Autodesk Fusion 360 part; units mm, degrees
note: some values were not read from the file. Chosen so that the rebuilt part matches the saved one: which bodies a step acts on. Set by a fixed rule: which sketch regions a step uses.
(part 2 of 5)
  constraint midpoint L119 L120.start
  constraint midpoint L117 L120.end
  constraint coincident L121 L124.start
  constraint coincident L122 L124.end
  constraint perpendicular L122 L124
  constraint midpoint L110 L169.start
  constraint midpoint L112 L169.end
  constraint symmetric A3.start L169 L12.end
  constraint symmetric L3.end L169 L11.end
  constraint symmetric L4.end L169 L10.end
  constraint symmetric L5.end L169 A8.start
  constraint symmetric L116.start L169 L170.end
  constraint symmetric L116.end L169 L173.start
  constraint symmetric L117.end L169 L172.start
  constraint symmetric L118.end L169 L170.start
  constraint symmetric L120.start L169 L171.start
  constraint symmetric L120.end L169 L171.end
  constraint symmetric L124.start L169 L218.start
  constraint symmetric L124.end L169 L218.end
  constraint symmetric L125.start L169 L176.start
  constraint symmetric L125.end L169 L176.end
  constraint symmetric L126.start L169 L175.start
  constraint symmetric L126.end L169 L174.start
  constraint symmetric L127.end L169 L174.end
  constraint symmetric L128.start L169 L180.start
  constraint symmetric L128.end L169 L180.end
  constraint symmetric L129.start L169 L179.start
  constraint symmetric L129.end L169 L178.start
  constraint symmetric L130.end L169 L178.end
  constraint symmetric L131.start L169 L184.start
  constraint symmetric L131.end L169 L184.end
  constraint symmetric L132.start L169 L183.start
  constraint symmetric L132.end L169 L182.start
  constraint symmetric L133.end L169 L182.end
  constraint symmetric L134.start L169 L188.start
  constraint symmetric L134.end L169 L188.end
  constraint symmetric L135.start L169 L187.start
  constraint symmetric L135.end L169 L186.start
  constraint symmetric L136.end L169 L186.end
  constraint symmetric L137.start L169 L191.start
  constraint symmetric L137.end L169 L191.end
  constraint symmetric L138.start L169 L192.start
  constraint symmetric L138.end L169 L190.start
  constraint symmetric L139.end L169 L190.end
  constraint symmetric L140.start L169 L196.start
  constraint symmetric L140.end L169 L196.end
  constraint symmetric L141.start L169 L195.start
  constraint symmetric L141.end L169 L194.start
  constraint symmetric L142.end L169 L194.end
  constraint symmetric L143.start L169 L199.start
  constraint symmetric L143.end L169 L199.end
  constraint symmetric L144.start L169 L200.start
  constraint symmetric L144.end L169 L198.start
  constraint symmetric L145.end L169 L198.end
  constraint symmetric L146.start L169 L204.start
  constraint symmetric L146.end L169 L204.end
  constraint symmetric L147.start L169 L203.start
  constraint symmetric L147.end L169 L202.start
  constraint symmetric L148.end L169 L202.end
  constraint symmetric L149.start L169 L208.start
  constraint symmetric L149.end L169 L208.end
  constraint symmetric L150.start L169 L207.start
  constraint symmetric L150.end L169 L206.start
  constraint symmetric L151.end L169 L206.end
  constraint symmetric L152.start L169 L212.start
  constraint symmetric L152.end L169 L212.end
  constraint symmetric L153.start L169 L211.start
  constraint symmetric L153.end L169 L210.start
  constraint symmetric L154.end L169 L210.end
  constraint symmetric L155.start L169 L215.start
  constraint symmetric L155.end L169 L215.end
  constraint symmetric L156.start L169 L216.start
  constraint symmetric L156.end L169 L214.start
  constraint symmetric L157.end L169 L214.end
  constraint symmetric L158.start L169 L177.start
  constraint symmetric L159.start L169 L181.start
  constraint symmetric L160.start L169 L185.start
  constraint symmetric L161.start L169 L189.start
  constraint symmetric L162.start L169 L193.start
  constraint symmetric L163.start L169 L197.start
  constraint symmetric L164.start L169 L201.start
  constraint symmetric L165.start L169 L205.start
  constraint symmetric L166.start L169 L209.start
  constraint symmetric L167.start L169 L213.start
  constraint symmetric L168.start L169 L217.start
  constraint concentric A56 A60
  constraint concentric A59 A61
  constraint equal A60 A61
  constraint concentric A68 A69
  constraint tangent A49 A68
  constraint vertical A49.centre A68.centre
  constraint coincident A49.centre L228.start
  constraint coincident A53.centre L228.end
  constraint symmetric A69 L228 A74
  constraint symmetric L228 A70 A75
  constraint symmetric L228 A72 A76
  constraint symmetric L228 A73 A77
  measures "d205" distance of L118 L120
  measures "d206" distance of L4 L124
  measures "d221" diameter of A60
  measures "d224" diameter of A68
  measures "d225" diameter of A69
extrude "Extrude1''" add sketch "Sketch2 (2)" along normal blind 3 separate body makes body 8 in component "led-pannel-frame_ply"
sketch "Sketch3 (2)" plane through (0, 0, -21) normal (0, 0, -1) x (1, 0, 0) in component "led-pannel-frame_ply"
  line L0 (110.5, 70.5) -> (105.75, 70.5)
  line L1 (105.75, 70.5) -> (105.75, 82.5)
  line L2 (105.75, 82.5) -> (110.5, 82.5)
  line L3 (110.5, 82.5) -> (110.5, 70.5)
  circle A0 centre (122.25, 61.125) radius 1.6
  line L4 (110.5, 87.5) -> (105.75, 87.5)
  line L5 (105.75, 87.5) -> (105.75, 99.5)
  line L6 (105.75, 99.5) -> (110.5, 99.5)
  line L7 (110.5, 99.5) -> (110.5, 87.5)
  line L8 (51, -124.5) -> (46.25, -124.5)
  line L9 (46.25, -124.5) -> (46.25, -112.5)
  line L10 (46.25, -112.5) -> (51, -112.5)
  line L11 (51, -112.5) -> (51, -124.5)
  circle A1 centre (0, 118.5) radius 7.5
  circle A2 centre (-61.125, -122.25) radius 1.6
  circle A3 centre (61.125, -122.25) radius 1.6
  circle A4 centre (122.25, -61.125) radius 1.6
  circle A5 centre (-61.125, 122.25) radius 1.6
  circle A6 centre (61.125, 122.25) radius 1.6
  circle A7 centre (-122.25, -61.125) radius 1.6
  circle A8 centre (-122.25, 61.125) radius 1.6
  circle A9 centre (-34, 123) radius 1.6
  circle A10 centre (-17, 123) radius 1.6
  circle A11 centre (17, 123) radius 1.6
  circle A12 centre (34, 123) radius 1.6
  circle A13 centre (-34, 114) radius 1.6
  circle A14 centre (17, 114) radius 1.6
  circle A15 centre (-17, 114) radius 1.6
  circle A16 centre (34, 114) radius 1.6
  circle A17 centre (-122.25, 122.25) radius 2.5
  circle A18 centre (-122.25, -122.25) radius 2.5
  line L12 (-105.75, -2.5) -> (-105.75, -14.5)
  line L13 (-105.75, -14.5) -> (-110.5, -14.5)
  line L14 (-110.5, -14.5) -> (-110.5, -2.5)
  line L15 (-110.5, -2.5) -> (-105.75, -2.5)
  line L16 (-105.75, -87.5) -> (-105.75, -99.5)
  line L17 (-105.75, -99.5) -> (-110.5, -99.5)
  line L18 (-110.5, -99.5) -> (-110.5, -87.5)
  line L19 (-110.5, -87.5) -> (-105.75, -87.5)
  circle A19 centre (122.25, 122.25) radius 2.5
  line L20 (-105.75, -19.5) -> (-105.75, -31.5)
  line L21 (-105.75, -31.5) -> (-110.5, -31.5)
  line L22 (-110.5, -31.5) -> (-110.5, -19.5)
  line L23 (-110.5, -19.5) -> (-105.75, -19.5)
  line L24 (-105.75, -36.5) -> (-105.75, -48.5)
  line L25 (-105.75, -48.5) -> (-110.5, -48.5)
  line L26 (-110.5, -48.5) -> (-110.5, -36.5)
  line L27 (-110.5, -36.5) -> (-105.75, -36.5)
  line L28 (-105.75, -53.5) -> (-105.75, -65.5)
  line L29 (-105.75, -65.5) -> (-110.5, -65.5)
  line L30 (-110.5, -65.5) -> (-110.5, -53.5)
  line L31 (-110.5, -53.5) -> (-105.75, -53.5)
  line L32 (-105.75, -70.5) -> (-105.75, -82.5)
  line L33 (-105.75, -82.5) -> (-110.5, -82.5)
  line L34 (-110.5, -82.5) -> (-110.5, -70.5)
  line L35 (-110.5, -70.5) -> (-105.75, -70.5)
  line L36 (-46.25, -112.5) -> (-46.25, -124.5)
  line L37 (-46.25, -124.5) -> (-51, -124.5)
  line L38 (-51, -124.5) -> (-51, -112.5)
  line L39 (-51, -112.5) -> (-46.25, -112.5)
  line L40 (-105.75, 14.5) -> (-105.75, 2.5)
  line L41 (-105.75, 2.5) -> (-110.5, 2.5)
  line L42 (-110.5, 2.5) -> (-110.5, 14.5)
  line L43 (-110.5, 14.5) -> (-105.75, 14.5)
  line L44 (-105.75, 31.5) -> (-105.75, 19.5)
  line L45 (-105.75, 19.5) -> (-110.5, 19.5)
  line L46 (-110.5, 19.5) -> (-110.5, 31.5)
  line L47 (-110.5, 31.5) -> (-105.75, 31.5)
  line L48 (-105.75, 48.5) -> (-105.75, 36.5)
  line L49 (-105.75, 36.5) -> (-110.5, 36.5)
  line L50 (-110.5, 36.5) -> (-110.5, 48.5)
  line L51 (-110.5, 48.5) -> (-105.75, 48.5)
  line L52 (-105.75, 65.5) -> (-105.75, 53.5)
  line L53 (-105.75, 53.5) -> (-110.5, 53.5)
  line L54 (-110.5, 53.5) -> (-110.5, 65.5)
  line L55 (-110.5, 65.5) -> (-105.75, 65.5)
  line L56 (-105.75, 82.5) -> (-105.75, 70.5)
  line L57 (-105.75, 70.5) -> (-110.5, 70.5)
  line L58 (-110.5, 70.5) -> (-110.5, 82.5)
  line L59 (-110.5, 82.5) -> (-105.75, 82.5)
  line L60 (-105.75, 99.5) -> (-105.75, 87.5)
  line L61 (-105.75, 87.5) -> (-110.5, 87.5)
  line L62 (-110.5, 87.5) -> (-110.5, 99.5)
  line L63 (-110.5, 99.5) -> (-105.75, 99.5)
  line L64 (110.5, -99.5) -> (105.75, -99.5)
  line L65 (105.75, -99.5) -> (105.75, -87.5)
  line L66 (105.75, -87.5) -> (110.5, -87.5)
  line L67 (110.5, -87.5) -> (110.5, -99.5)
  line L68 (110.5, -82.5) -> (105.75, -82.5)
  line L69 (105.75, -82.5) -> (105.75, -70.5)
  line L70 (105.75, -70.5) -> (110.5, -70.5)
  line L71 (110.5, -70.5) -> (110.5, -82.5)
  line L72 (110.5, -65.5) -> (105.75, -65.5)
  line L73 (105.75, -65.5) -> (105.75, -53.5)
  line L74 (105.75, -53.5) -> (110.5, -53.5)
  line L75 (110.5, -53.5) -> (110.5, -65.5)
  line L76 (110.5, -48.5) -> (105.75, -48.5)
  line L77 (105.75, -48.5) -> (105.75, -36.5)
  line L78 (105.75, -36.5) -> (110.5, -36.5)
  line L79 (110.5, -36.5) -> (110.5, -48.5)
  line L80 (110.5, -31.5) -> (105.75, -31.5)
  line L81 (105.75, -31.5) -> (105.75, -19.5)
  line L82 (105.75, -19.5) -> (110.5, -19.5)
  line L83 (110.5, -19.5) -> (110.5, -31.5)
  line L84 (110.5, 36.5) -> (105.75, 36.5)
  line L85 (105.75, 36.5) -> (105.75, 48.5)
  line L86 (105.75, 48.5) -> (110.5, 48.5)
  line L87 (110.5, 48.5) -> (110.5, 36.5)
  line L88 (110.5, -14.5) -> (105.75, -14.5)
  line L89 (105.75, -14.5) -> (105.75, -2.5)
  line L90 (105.75, -2.5) -> (110.5, -2.5)
  line L91 (110.5, -2.5) -> (110.5, -14.5)
  line L92 (110.5, 53.5) -> (105.75, 53.5)
  line L93 (105.75, 53.5) -> (105.75, 65.5)
  line L94 (105.75, 65.5) -> (110.5, 65.5)
  line L95 (110.5, 65.5) -> (110.5, 53.5)
  line L96 (110.5, 2.5) -> (105.75, 2.5)
  line L97 (105.75, 2.5) -> (105.75, 14.5)
  line L98 (105.75, 14.5) -> (110.5, 14.5)
  line L99 (110.5, 14.5) -> (110.5, 2.5)
  line L100 (110.5, 19.5) -> (105.75, 19.5)
  line L101 (105.75, 19.5) -> (105.75, 31.5)
  line L102 (105.75, 31.5) -> (110.5, 31.5)
  line L103 (110.5, 31.5) -> (110.5, 19.5)
  circle A20 centre (122.25, -122.25) radius 2.5
  arc A21 (-129.75, -122.25) -> (-122.25, -129.75) centre (-122.25, -122.25) ccw
  line L104 (-122.25, -129.75) -> (122.25, -129.75)
  arc A22 (122.25, -129.75) -> (129.75, -122.25) centre (122.25, -122.25) ccw
  line L105 (129.75, -122.25) -> (129.75, 122.25)
  arc A23 (129.75, 122.25) -> (122.25, 129.75) centre (122.25, 122.25) ccw
  line L106 (122.25, 129.75) -> (-122.25, 129.75)
  arc A24 (-122.25, 129.75) -> (-129.75, 122.25) centre (-122.25, 122.25) ccw
  line L107 (-129.75, 122.25) -> (-129.75, -122.25)
sketch "Sketch1 (2)" plane through (0, 0, -18) normal (0, 0, 1) x (-1, 0, 0) in component "grid_3d"
  line L0 (-105.75, 70.5) -> (-110.5, 70.5)
  line L1 (-110.5, 70.5) -> (-110.5, 82.5)
  line L2 (-110.5, 82.5) -> (-105.75, 82.5)
  line L3 (-105.75, 82.5) -> (-105.75, 70.5)
  circle A0 centre (-122.25, 61.125) radius 1.6
  line L4 (-105.75, 87.5) -> (-110.5, 87.5)
  line L5 (-110.5, 87.5) -> (-110.5, 99.5)
  line L6 (-110.5, 99.5) -> (-105.75, 99.5)
  line L7 (-105.75, 99.5) -> (-105.75, 87.5)
  line L8 (-46.25, -124.5) -> (-51, -124.5)
  line L9 (-51, -124.5) -> (-51, -112.5)
  line L10 (-51, -112.5) -> (-46.25, -112.5)
  line L11 (-46.25, -112.5) -> (-46.25, -124.5)
  circle A1 centre (0, 118.5) radius 7.5
  circle A2 centre (61.125, -122.25) radius 1.6
  circle A3 centre (-61.125, -122.25) radius 1.6
  circle A4 centre (-122.25, -61.125) radius 1.6
  circle A5 centre (61.125, 122.25) radius 1.6
  circle A6 centre (-61.125, 122.25) radius 1.6
  circle A7 centre (122.25, -61.125) radius 1.6
  circle A8 centre (122.25, 61.125) radius 1.6
  circle A9 centre (34, 123) radius 1.6
  circle A10 centre (17, 123) radius 1.6
  circle A11 centre (-17, 123) radius 1.6
  circle A12 centre (-34, 123) radius 1.6
  circle A13 centre (34, 114) radius 1.6
  circle A14 centre (-17, 114) radius 1.6
  circle A15 centre (17, 114) radius 1.6
  circle A16 centre (-34, 114) radius 1.6
  circle A17 centre (122.25, 122.25) radius 2.5
  circle A18 centre (122.25, -122.25) radius 2.5
  line L12 (105.75, -14.5) -> (105.75, -2.5)
  line L13 (105.75, -2.5) -> (110.5, -2.5)
  line L14 (110.5, -2.5) -> (110.5, -14.5)
  line L15 (110.5, -14.5) -> (105.75, -14.5)
  line L16 (105.75, -99.5) -> (105.75, -87.5)
  line L17 (105.75, -87.5) -> (110.5, -87.5)
  line L18 (110.5, -87.5) -> (110.5, -99.5)
  line L19 (110.5, -99.5) -> (105.75, -99.5)
  circle A19 centre (-122.25, 122.25) radius 2.5
  line L20 (105.75, -31.5) -> (105.75, -19.5)
  line L21 (105.75, -19.5) -> (110.5, -19.5)
  line L22 (110.5, -19.5) -> (110.5, -31.5)
  line L23 (110.5, -31.5) -> (105.75, -31.5)
  line L24 (105.75, -48.5) -> (105.75, -36.5)
  line L25 (105.75, -36.5) -> (110.5, -36.5)
  line L26 (110.5, -36.5) -> (110.5, -48.5)
  line L27 (110.5, -48.5) -> (105.75, -48.5)
  line L28 (105.75, -65.5) -> (105.75, -53.5)
  line L29 (105.75, -53.5) -> (110.5, -53.5)
  line L30 (110.5, -53.5) -> (110.5, -65.5)
  line L31 (110.5, -65.5) -> (105.75, -65.5)
  line L32 (105.75, -82.5) -> (105.75, -70.5)
  line L33 (105.75, -70.5) -> (110.5, -70.5)
  line L34 (110.5, -70.5) -> (110.5, -82.5)
  line L35 (110.5, -82.5) -> (105.75, -82.5)
  line L36 (46.25, -124.5) -> (46.25, -112.5)
  line L37 (46.25, -112.5) -> (51, -112.5)
  line L38 (51, -112.5) -> (51, -124.5)
  line L39 (51, -124.5) -> (46.25, -124.5)
  line L40 (105.75, 2.5) -> (105.75, 14.5)
  line L41 (105.75, 14.5) -> (110.5, 14.5)
  line L42 (110.5, 14.5) -> (110.5, 2.5)
  line L43 (110.5, 2.5) -> (105.75, 2.5)
  line L44 (105.75, 19.5) -> (105.75, 31.5)
  line L45 (105.75, 31.5) -> (110.5, 31.5)
  line L46 (110.5, 31.5) -> (110.5, 19.5)
  line L47 (110.5, 19.5) -> (105.75, 19.5)
  line L48 (105.75, 36.5) -> (105.75, 48.5)
  line L49 (105.75, 48.5) -> (110.5, 48.5)
  line L50 (110.5, 48.5) -> (110.5, 36.5)
  line L51 (110.5, 36.5) -> (105.75, 36.5)
  line L52 (105.75, 53.5) -> (105.75, 65.5)
  line L53 (105.75, 65.5) -> (110.5, 65.5)
  line L54 (110.5, 65.5) -> (110.5, 53.5)
  line L55 (110.5, 53.5) -> (105.75, 53.5)
  line L56 (105.75, 70.5) -> (105.75, 82.5)
  line L57 (105.75, 82.5) -> (110.5, 82.5)
  line L58 (110.5, 82.5) -> (110.5, 70.5)
  line L59 (110.5, 70.5) -> (105.75, 70.5)
  line L60 (105.75, 87.5) -> (105.75, 99.5)
  line L61 (105.75, 99.5) -> (110.5, 99.5)
  line L62 (110.5, 99.5) -> (110.5, 87.5)
  line L63 (110.5, 87.5) -> (105.75, 87.5)
  line L64 (-105.75, -99.5) -> (-110.5, -99.5)
  line L65 (-110.5, -99.5) -> (-110.5, -87.5)
  line L66 (-110.5, -87.5) -> (-105.75, -87.5)
  line L67 (-105.75, -87.5) -> (-105.75, -99.5)
  line L68 (-105.75, -82.5) -> (-110.5, -82.5)
  line L69 (-110.5, -82.5) -> (-110.5, -70.5)
  line L70 (-110.5, -70.5) -> (-105.75, -70.5)
  line L71 (-105.75, -70.5) -> (-105.75, -82.5)
  line L72 (-105.75, -65.5) -> (-110.5, -65.5)
  line L73 (-110.5, -65.5) -> (-110.5, -53.5)
  line L74 (-110.5, -53.5) -> (-105.75, -53.5)
  line L75 (-105.75, -53.5) -> (-105.75, -65.5)
  line L76 (-105.75, -48.5) -> (-110.5, -48.5)
  line L77 (-110.5, -48.5) -> (-110.5, -36.5)
  line L78 (-110.5, -36.5) -> (-105.75, -36.5)
  line L79 (-105.75, -36.5) -> (-105.75, -48.5)
  line L80 (-105.75, -31.5) -> (-110.5, -31.5)
  line L81 (-110.5, -31.5) -> (-110.5, -19.5)
  line L82 (-110.5, -19.5) -> (-105.75, -19.5)
  line L83 (-105.75, -19.5) -> (-105.75, -31.5)
  line L84 (-105.75, 36.5) -> (-110.5, 36.5)
  line L85 (-110.5, 36.5) -> (-110.5, 48.5)
  line L86 (-110.5, 48.5) -> (-105.75, 48.5)
  line L87 (-105.75, 48.5) -> (-105.75, 36.5)
  line L88 (-105.75, -14.5) -> (-110.5, -14.5)
  line L89 (-110.5, -14.5) -> (-110.5, -2.5)
  line L90 (-110.5, -2.5) -> (-105.75, -2.5)
  line L91 (-105.75, -2.5) -> (-105.75, -14.5)
  line L92 (-105.75, 53.5) -> (-110.5, 53.5)
  line L93 (-110.5, 53.5) -> (-110.5, 65.5)
  line L94 (-110.5, 65.5) -> (-105.75, 65.5)
  line L95 (-105.75, 65.5) -> (-105.75, 53.5)
  line L96 (-105.75, 2.5) -> (-110.5, 2.5)
  line L97 (-110.5, 2.5) -> (-110.5, 14.5)
  line L98 (-110.5, 14.5) -> (-105.75, 14.5)
  line L99 (-105.75, 14.5) -> (-105.75, 2.5)
  line L100 (-105.75, 19.5) -> (-110.5, 19.5)
  line L101 (-110.5, 19.5) -> (-110.5, 31.5)
  line L102 (-110.5, 31.5) -> (-105.75, 31.5)
  line L103 (-105.75, 31.5) -> (-105.75, 19.5)
  circle A20 centre (-122.25, -122.25) radius 2.5
  arc A21 (122.25, -129.75) -> (129.75, -122.25) centre (122.25, -122.25) ccw
  line L104 (129.75, -122.25) -> (129.75, 122.25)
  arc A22 (129.75, 122.25) -> (122.25, 129.75) centre (122.25, 122.25) ccw
  line L105 (122.25, 129.75) -> (-122.25, 129.75)
  arc A23 (-122.25, 129.75) -> (-129.75, 122.25) centre (-122.25, 122.25) ccw
  line L106 (-129.75, 122.25) -> (-129.75, -122.25)
  arc A24 (-129.75, -122.25) -> (-122.25, -129.75) centre (-122.25, -122.25) ccw
  line L107 (-122.25, -129.75) -> (122.25, -129.75)
  arc A25 (-129.75, 69.625) -> (-128.75, 68.625) centre (-128.75, 69.625) ccw
  line L108 (-129.75, 69.625) -> (-129.75, 116.02505)
  arc A26 (-128.027778, 116.716711) -> (-129.75, 116.02505) centre (-128.75, 116.02505) ccw
  arc A27 (-128.027778, 116.716711) -> (-117.256712, 115.999634) centre (-122.25, 122.25) ccw
  arc A28 (-115.925445, 115.925445) -> (-117.256712, 115.999634) centre (-116.632551, 115.218338) ccw
  line L109 (-115.925445, 115.925445) -> (-101.292893, 101.292893)
  arc A29 (-101, 100.585786) -> (-101.292893, 101.292893) centre (-102, 100.585786) ccw
  line L110 (-101, 100.585786) -> (-101, 99.5)
  line L111 (-101, 99.5) -> (-110.5, 99.5)
  line L112 (-110.5, 99.5) -> (-110.5, 87.5)
  line L113 (-110.5, 87.5) -> (-101, 87.5)
  line L114 (-101, 87.5) -> (-101, 87)
  arc A30 (-102, 86) -> (-101, 87) centre (-102, 87) ccw
  line L115 (-102, 86) -> (-108.5, 86)
  line L116 (-108.5, 86) -> (-108.5, 84)
  line L117 (-108.5, 84) -> (-102, 84)
  arc A31 (-101, 83) -> (-102, 84) centre (-102, 83) ccw
  line L118 (-101, 83) -> (-101, 82.5)
  line L119 (-101, 82.5) -> (-110.5, 82.5)
  line L120 (-110.5, 82.5) -> (-110.5, 70.5)
  line L121 (-110.5, 70.5) -> (-101, 70.5)
  line L122 (-101, 70.5) -> (-101, 70)
  arc A32 (-102, 69) -> (-101, 70) centre (-102, 70) ccw
  line L123 (-102, 69) -> (-108.5, 69)
  line L124 (-108.5, 69) -> (-108.5, 67)
  line L125 (-108.5, 67) -> (-102, 67)
  arc A33 (-101, 66) -> (-102, 67) centre (-102, 66) ccw
  line L126 (-101, 66) -> (-101, 65.5)
  line L127 (-101, 65.5) -> (-110.5, 65.5)
  line L128 (-110.5, 65.5) -> (-110.5, 53.5)
  line L129 (-110.5, 53.5) -> (-101, 53.5)
  line L130 (-101, 53.5) -> (-101, 53)
  arc A34 (-102, 52) -> (-101, 53) centre (-102, 53) ccw
  line L131 (-102, 52) -> (-108.5, 52)
  line L132 (-108.5, 52) -> (-108.5, 50)
  line L133 (-108.5, 50) -> (-102, 50)
  arc A35 (-101, 49) -> (-102, 50) centre (-102, 49) ccw
  line L134 (-101, 49) -> (-101, 48.5)
  line L135 (-101, 48.5) -> (-110.5, 48.5)
  line L136 (-110.5, 48.5) -> (-110.5, 36.5)
  line L137 (-110.5, 36.5) -> (-101, 36.5)
  line L138 (-101, 36.5) -> (-101, 36)
  arc A36 (-102, 35) -> (-101, 36) centre (-102, 36) ccw
  line L139 (-102, 35) -> (-108.5, 35)
  line L140 (-108.5, 35) -> (-108.5, 33)
  line L141 (-108.5, 33) -> (-102, 33)
  arc A37 (-101, 32) -> (-102, 33) centre (-102, 32) ccw
  line L142 (-101, 32) -> (-101, 31.5)
  line L143 (-101, 31.5) -> (-110.5, 31.5)
  line L144 (-110.5, 31.5) -> (-110.5, 19.5)
  line L145 (-110.5, 19.5) -> (-101, 19.5)
  line L146 (-101, 19.5) -> (-101, 19)
  arc A38 (-102, 18) -> (-101, 19) centre (-102, 19) ccw
  line L147 (-102, 18) -> (-108.5, 18)
  line L148 (-108.5, 18) -> (-108.5, 16)
  line L149 (-108.5, 16) -> (-102, 16)
  arc A39 (-101, 15) -> (-102, 16) centre (-102, 15) ccw
  line L150 (-101, 15) -> (-101, 14.5)
  line L151 (-101, 14.5) -> (-110.5, 14.5)
  line L152 (-110.5, 14.5) -> (-110.5, 2.5)
  line L153 (-110.5, 2.5) -> (-101, 2.5)
  line L154 (-101, 2.5) -> (-101, 2)
  arc A40 (-102, 1) -> (-101, 2) centre (-102, 2) ccw
  line L155 (-102, 1) -> (-108.5, 1)
  line L156 (-108.5, 1) -> (-108.5, -1)
  line L157 (-108.5, -1) -> (-102, -1)
  arc A41 (-101, -2) -> (-102, -1) centre (-102, -2) ccw
  line L158 (-101, -2) -> (-101, -2.5)
  line L159 (-101, -2.5) -> (-110.5, -2.5)
  line L160 (-110.5, -2.5) -> (-110.5, -14.5)
  line L161 (-110.5, -14.5) -> (-101, -14.5)
  line L162 (-101, -14.5) -> (-101, -15)
  arc A42 (-102, -16) -> (-101, -15) centre (-102, -15) ccw
  line L163 (-102, -16) -> (-108.5, -16)
  line L164 (-108.5, -16) -> (-108.5, -18)
  line L165 (-108.5, -18) -> (-102, -18)
  arc A43 (-101, -19) -> (-102, -18) centre (-102, -19) ccw
  line L166 (-101, -19) -> (-101, -19.5)
  line L167 (-101, -19.5) -> (-110.5, -19.5)
  line L168 (-110.5, -19.5) -> (-110.5, -31.5)
  line L169 (-110.5, -31.5) -> (-101, -31.5)
  line L170 (-101, -31.5) -> (-101, -32)
  arc A44 (-102, -33) -> (-101, -32) centre (-102, -32) ccw
  line L171 (-102, -33) -> (-108.5, -33)
  line L172 (-108.5, -33) -> (-108.5, -35)
  line L173 (-108.5, -35) -> (-102, -35)
  arc A45 (-101, -36) -> (-102, -35) centre (-102, -36) ccw
  line L174 (-101, -36) -> (-101, -36.5)
  line L175 (-101, -36.5) -> (-110.5, -36.5)
  line L176 (-110.5, -36.5) -> (-110.5, -48.5)
  line L177 (-110.5, -48.5) -> (-101, -48.5)
  line L178 (-101, -48.5) -> (-101, -49)
  arc A46 (-102, -50) -> (-101, -49) centre (-102, -49) ccw
  line L179 (-102, -50) -> (-108.5, -50)
  line L180 (-108.5, -50) -> (-108.5, -52)
  line L181 (-108.5, -52) -> (-102, -52)
  arc A47 (-101, -53) -> (-102, -52) centre (-102, -53) ccw
  line L182 (-101, -53) -> (-101, -53.5)
  line L183 (-101, -53.5) -> (-110.5, -53.5)
  line L184 (-110.5, -53.5) -> (-110.5, -65.5)
  line L185 (-110.5, -65.5) -> (-101, -65.5)
  line L186 (-101, -65.5) -> (-101, -66)
  arc A48 (-102, -67) -> (-101, -66) centre (-102, -66) ccw
  line L187 (-102, -67) -> (-108.5, -67)
  line L188 (-108.5, -67) -> (-108.5, -69)
  line L189 (-108.5, -69) -> (-102, -69)
  arc A49 (-101, -70) -> (-102, -69) centre (-102, -70) ccw
  line L190 (-101, -70) -> (-101, -70.5)
  line L191 (-101, -70.5) -> (-110.5, -70.5)
  line L192 (-110.5, -70.5) -> (-110.5, -82.5)
  line L193 (-110.5, -82.5) -> (-101, -82.5)
  line L194 (-101, -82.5) -> (-101, -83)
  arc A50 (-102, -84) -> (-101, -83) centre (-102, -83) ccw
  line L195 (-102, -84) -> (-108.5, -84)
  line L196 (-108.5, -84) -> (-108.5, -86)
  line L197 (-108.5, -86) -> (-102, -86)
  arc A51 (-101, -87) -> (-102, -86) centre (-102, -87) ccw
  line L198 (-101, -87) -> (-101, -87.5)
  line L199 (-101, -87.5) -> (-110.5, -87.5)
  line L200 (-110.5, -87.5) -> (-110.5, -99.5)
  line L201 (-110.5, -99.5) -> (-101, -99.5)
  line L202 (-101, -99.5) -> (-101, -100.585786)
  arc A52 (-101.292893, -101.292893) -> (-101, -100.585786) centre (-102, -100.585786) ccw
  line L203 (-101.292893, -101.292893) -> (-116.946699, -116.946699)
  arc A53 (-129.75, -122.25) -> (-116.946699, -116.946699) centre (-122.25, -122.25) ccw
  line L204 (-129.75, -122.25) -> (-129.75, -69.625)
  arc A54 (-128.75, -68.625) -> (-129.75, -69.625) centre (-128.75, -69.625) ccw
  line L205 (-128.75, -68.625) -> (-122.25, -68.625)
  arc A55 (-122.25, -68.625) -> (-122.25, -53.625) centre (-122.25, -61.125) ccw
  line L206 (-122.25, -53.625) -> (-128.75, -53.625)
  arc A56 (-129.75, -52.625) -> (-128.75, -53.625) centre (-128.75, -52.625) ccw
  line L207 (-129.75, -52.625) -> (-129.75, 52.625)
  arc A57 (-128.75, 53.625) -> (-129.75, 52.625) centre (-128.75, 52.625) ccw
  line L208 (-128.75, 53.625) -> (-122.25, 53.625)
  arc A58 (-122.25, 53.625) -> (-122.25, 68.625) centre (-122.25, 61.125) ccw
  line L209 (-122.25, 68.625) -> (-128.75, 68.625)
  circle A59 centre (-122.25, -122.25) radius 2.5
  line L210 (-124.5, 12.5) -> (-124.5, 4.5)
  arc A60 (-124.5, 4.5) -> (-124.5, -4.5) centre (-118.5, 0) ccw
  line L211 (-124.5, -4.5) -> (-124.5, -12.5)
  arc A61 (-124.5, -12.5) -> (-124.5, -21.5) centre (-118.5, -17) ccw
  line L212 (-124.5, -21.5) -> (-124.5, -29.5)
  arc A62 (-124.5, -29.5) -> (-124.5, -38.5) centre (-118.5, -34) ccw
  line L213 (-124.5, -38.5) -> (-124.5, -51)
  line L214 (-124.5, -51) -> (-112.5, -51)
  line L215 (-112.5, -51) -> (-112.5, -38.5)
  arc A63 (-112.5, -38.5) -> (-112.5, -29.5) centre (-118.5, -34) ccw
  line L216 (-112.5, -29.5) -> (-112.5, -21.5)
  arc A64 (-112.5, -21.5) -> (-112.5, -12.5) centre (-118.5, -17) ccw
  line L217 (-112.5, -12.5) -> (-112.5, -4.5)
  arc A65 (-112.5, -4.5) -> (-112.5, 4.5) centre (-118.5, 0) ccw
  line L218 (-112.5, 4.5) -> (-112.5, 12.5)
  arc A66 (-112.5, 12.5) -> (-112.5, 21.5) centre (-118.5, 17) ccw
  line L219 (-112.5, 21.5) -> (-112.5, 29.5)
  arc A67 (-112.5, 29.5) -> (-112.5, 38.5) centre (-118.5, 34) ccw
  line L220 (-112.5, 38.5) -> (-112.5, 51)
  line L221 (-112.5, 51) -> (-124.5, 51)
  line L222 (-124.5, 51) -> (-124.5, 38.5)
  arc A68 (-124.5, 38.5) -> (-124.5, 29.5) centre (-118.5, 34) ccw
  line L223 (-124.5, 29.5) -> (-124.5, 21.5)
  arc A69 (-124.5, 21.5) -> (-124.5, 12.5) centre (-118.5, 17) ccw
  arc A70 (129.75, -69.625) -> (128.75, -68.625) centre (128.75, -69.625) ccw
  line L224 (129.75, -69.625) -> (129.75, -116.02505)
  arc A71 (128.027778, -116.716711) -> (129.75, -116.02505) centre (128.75, -116.02505) ccw
  arc A72 (128.027778, -116.716711) -> (117.256712, -115.999634) centre (122.25, -122.25) ccw
  arc A73 (115.925445, -115.925445) -> (117.256712, -115.999634) centre (116.632551, -115.218338) ccw
  line L225 (115.925445, -115.925445) -> (101.292893, -101.292893)
  arc A74 (101, -100.585786) -> (101.292893, -101.292893) centre (102, -100.585786) ccw
  line L226 (101, -100.585786) -> (101, -99.5)
  line L227 (101, -99.5) -> (110.5, -99.5)
  line L228 (110.5, -99.5) -> (110.5, -87.5)
  line L229 (110.5, -87.5) -> (101, -87.5)
  line L230 (101, -87.5) -> (101, -87)
  arc A75 (102, -86) -> (101, -87) centre (102, -87) ccw
  line L231 (102, -86) -> (108.5, -86)
  line L232 (108.5, -86) -> (108.5, -84)
  line L233 (108.5, -84) -> (102, -84)
  arc A76 (101, -83) -> (102, -84) centre (102, -83) ccw
  line L234 (101, -83) -> (101, -82.5)
  line L235 (101, -82.5) -> (110.5, -82.5)
  line L236 (110.5, -82.5) -> (110.5, -70.5)
  line L237 (110.5, -70.5) -> (101, -70.5)
  line L238 (101, -70.5) -> (101, -70)
  arc A77 (102, -69) -> (101, -70) centre (102, -70) ccw
  line L239 (102, -69) -> (108.5, -69)
  line L240 (108.5, -69) -> (108.5, -67)
  line L241 (108.5, -67) -> (102, -67)
  arc A78 (101, -66) -> (102, -67) centre (102, -66) ccw
  line L242 (101, -66) -> (101, -65.5)
  line L243 (101, -65.5) -> (110.5, -65.5)
  line L244 (110.5, -65.5) -> (110.5, -53.5)
  line L245 (110.5, -53.5) -> (101, -53.5)
  line L246 (101, -53.5) -> (101, -53)
  arc A79 (102, -52) -> (101, -53) centre (102, -53) ccw
  line L247 (102, -52) -> (108.5, -52)
  line L248 (108.5, -52) -> (108.5, -50)
  line L249 (108.5, -50) -> (102, -50)
  arc A80 (101, -49) -> (102, -50) centre (102, -49) ccw
  line L250 (101, -49) -> (101, -48.5)
  line L251 (101, -48.5) -> (110.5, -48.5)
  line L252 (110.5, -48.5) -> (110.5, -36.5)
  line L253 (110.5, -36.5) -> (101, -36.5)
  line L254 (101, -36.5) -> (101, -36)
  arc A81 (102, -35) -> (101, -36) centre (102, -36) ccw
  line L255 (102, -35) -> (108.5, -35)
  line L256 (108.5, -35) -> (108.5, -33)
  line L257 (108.5, -33) -> (102, -33)
  arc A82 (101, -32) -> (102, -33) centre (102, -32) ccw
  line L258 (101, -32) -> (101, -31.5)
  line L259 (101, -31.5) -> (110.5, -31.5)
  line L260 (110.5, -31.5) -> (110.5, -19.5)
  line L261 (110.5, -19.5) -> (101, -19.5)
  line L262 (101, -19.5) -> (101, -19)
  arc A83 (102, -18) -> (101, -19) centre (102, -19) ccw
  line L263 (102, -18) -> (108.5, -18)
  line L264 (108.5, -18) -> (108.5, -16)
  line L265 (108.5, -16) -> (102, -16)
  arc A84 (101, -15) -> (102, -16) centre (102, -15) ccw
  line L266 (101, -15) -> (101, -14.5)
  line L267 (101, -14.5) -> (110.5, -14.5)
  line L268 (110.5, -14.5) -> (110.5, -2.5)
  line L269 (110.5, -2.5) -> (101, -2.5)
  line L270 (101, -2.5) -> (101, -2)
  arc A85 (102, -1) -> (101, -2) centre (102, -2) ccw
  line L271 (102, -1) -> (108.5, -1)
  line L272 (108.5, -1) -> (108.5, 1)
  line L273 (108.5, 1) -> (102, 1)
  arc A86 (101, 2) -> (102, 1) centre (102, 2) ccw
  line L274 (101, 2) -> (101, 2.5)
  line L275 (101, 2.5) -> (110.5, 2.5)
  line L276 (110.5, 2.5) -> (110.5, 14.5)
  line L277 (110.5, 14.5) -> (101, 14.5)
  line L278 (101, 14.5) -> (101, 15)
  arc A87 (102, 16) -> (101, 15) centre (102, 15) ccw
  line L279 (102, 16) -> (108.5, 16)
  line L280 (108.5, 16) -> (108.5, 18)
  line L281 (108.5, 18) -> (102, 18)
  arc A88 (101, 19) -> (102, 18) centre (102, 19) ccw
  line L282 (101, 19) -> (101, 19.5)
  line L283 (101, 19.5) -> (110.5, 19.5)
  line L284 (110.5, 19.5) -> (110.5, 31.5)
  line L285 (110.5, 31.5) -> (101, 31.5)
  line L286 (101, 31.5) -> (101, 32)
  arc A89 (102, 33) -> (101, 32) centre (102, 32) ccw
  line L287 (102, 33) -> (108.5, 33)
  line L288 (108.5, 33) -> (108.5, 35)
  line L289 (108.5, 35) -> (102, 35)
  arc A90 (101, 36) -> (102, 35) centre (102, 36) ccw
  line L290 (101, 36) -> (101, 36.5)
  line L291 (101, 36.5) -> (110.5, 36.5)
  line L292 (110.5, 36.5) -> (110.5, 48.5)
  line L293 (110.5, 48.5) -> (101, 48.5)
  line L294 (101, 48.5) -> (101, 49)
  arc A91 (102, 50) -> (101, 49) centre (102, 49) ccw
  line L295 (102, 50) -> (108.5, 50)
  line L296 (108.5, 50) -> (108.5, 52)
  line L297 (108.5, 52) -> (102, 52)
  arc A92 (101, 53) -> (102, 52) centre (102, 53) ccw
  line L298 (101, 53) -> (101, 53.5)
  line L299 (101, 53.5) -> (110.5, 53.5)
  line L300 (110.5, 53.5) -> (110.5, 65.5)
  line L301 (110.5, 65.5) -> (101, 65.5)
  line L302 (101, 65.5) -> (101, 66)
  arc A93 (102, 67) -> (101, 66) centre (102, 66) ccw
  line L303 (102, 67) -> (108.5, 67)
  line L304 (108.5, 67) -> (108.5, 69)
  line L305 (108.5, 69) -> (102, 69)
  arc A94 (101, 70) -> (102, 69) centre (102, 70) ccw
  line L306 (101, 70) -> (101, 70.5)
  line L307 (101, 70.5) -> (110.5, 70.5)
  line L308 (110.5, 70.5) -> (110.5, 82.5)
  line L309 (110.5, 82.5) -> (101, 82.5)
  line L310 (101, 82.5) -> (101, 83)
  arc A95 (102, 84) -> (101, 83) centre (102, 83) ccw
  line L311 (102, 84) -> (108.5, 84)
  line L312 (108.5, 84) -> (108.5, 86)
  line L313 (108.5, 86) -> (102, 86)
  arc A96 (101, 87) -> (102, 86) centre (102, 87) ccw
  line L314 (101, 87) -> (101, 87.5)
  line L315 (101, 87.5) -> (110.5, 87.5)
  line L316 (110.5, 87.5) -> (110.5, 99.5)
  line L317 (110.5, 99.5) -> (101, 99.5)
  line L318 (101, 99.5) -> (101, 100.585786)
  arc A97 (101.292893, 101.292893) -> (101, 100.585786) centre (102, 100.585786) ccw
  line L319 (101.292893, 101.292893) -> (116.946699, 116.946699)
  arc A98 (129.75, 122.25) -> (116.946699, 116.946699) centre (122.25, 122.25) ccw
  line L320 (129.75, 122.25) -> (129.75, 69.625)
  arc A99 (128.75, 68.625) -> (129.75, 69.625) centre (128.75, 69.625) ccw
  line L321 (128.75, 68.625) -> (122.25, 68.625)
  arc A100 (122.25, 68.625) -> (122.25, 53.625) centre (122.25, 61.125) ccw
  line L322 (122.25, 53.625) -> (128.75, 53.625)
  arc A101 (129.75, 52.625) -> (128.75, 53.625) centre (128.75, 52.625) ccw
  line L323 (129.75, 52.625) -> (129.75, -52.625)
  arc A102 (128.75, -53.625) -> (129.75, -52.625) centre (128.75, -52.625) ccw
  line L324 (128.75, -53.625) -> (122.25, -53.625)
  arc A103 (122.25, -53.625) -> (122.25, -68.625) centre (122.25, -61.125) ccw
  line L325 (122.25, -68.625) -> (128.75, -68.625)
  circle A104 centre (122.25, 122.25) radius 2.5
  line L326 (124.5, -12.5) -> (124.5, -4.5)
  arc A105 (124.5, -4.5) -> (124.5, 4.5) centre (118.5, 0) ccw
  line L327 (124.5, 4.5) -> (124.5, 12.5)
  arc A106 (124.5, 12.5) -> (124.5, 21.5) centre (118.5, 17) ccw
  line L328 (124.5, 21.5) -> (124.5, 29.5)
  arc A107 (124.5, 29.5) -> (124.5, 38.5) centre (118.5, 34) ccw
  line L329 (124.5, 38.5) -> (124.5, 51)
  line L330 (124.5, 51) -> (112.5, 51)
  line L331 (112.5, 51) -> (112.5, 38.5)
  arc A108 (112.5, 38.5) -> (112.5, 29.5) centre (118.5, 34) ccw
  line L332 (112.5, 29.5) -> (112.5, 21.5)
  arc A109 (112.5, 21.5) -> (112.5, 12.5) centre (118.5, 17) ccw
  line L333 (112.5, 12.5) -> (112.5, 4.5)
  arc A110 (112.5, 4.5) -> (112.5, -4.5) centre (118.5, 0) ccw
  line L334 (112.5, -4.5) -> (112.5, -12.5)
  arc A111 (112.5, -12.5) -> (112.5, -21.5) centre (118.5, -17) ccw
  line L335 (112.5, -21.5) -> (112.5, -29.5)
  arc A112 (112.5, -29.5) -> (112.5, -38.5) centre (118.5, -34) ccw
  line L336 (112.5, -38.5) -> (112.5, -51)
  line L337 (112.5, -51) -> (124.5, -51)
  line L338 (124.5, -51) -> (124.5, -38.5)
  arc A113 (124.5, -38.5) -> (124.5, -29.5) centre (118.5, -34) ccw
  line L339 (124.5, -29.5) -> (124.5, -21.5)
  arc A114 (124.5, -21.5) -> (124.5, -12.5) centre (118.5, -17) ccw
  arc A115 (-69.625, -129.75) -> (-68.625, -128.75) centre (-69.625, -128.75) ccw
  line L340 (-69.625, -129.75) -> (-116.02505, -129.75)
  arc A116 (-116.716711, -128.027778) -> (-116.02505, -129.75) centre (-116.02505, -128.75) ccw
  arc A117 (-116.716711, -128.027778) -> (-115.999634, -117.256712) centre (-122.25, -122.25) ccw
  arc A118 (-115.925445, -115.925445) -> (-115.999634, -117.256712) centre (-115.218338, -116.632551) ccw
  line L341 (-115.925445, -115.925445) -> (-101.292893, -101.292893)
  arc A119 (-100.585786, -101) -> (-101.292893, -101.292893) centre (-100.585786, -102) ccw
  line L342 (-100.585786, -101) -> (-99.5, -101)
  line L343 (-99.5, -101) -> (-99.5, -110.5)
  line L344 (-99.5, -110.5) -> (-87.5, -110.5)
  line L345 (-87.5, -110.5) -> (-87.5, -101)
  line L346 (-87.5, -101) -> (-87, -101)
  arc A120 (-86, -102) -> (-87, -101) centre (-87, -102) ccw
  line L347 (-86, -102) -> (-86, -108.5)
  line L348 (-86, -108.5) -> (-84, -108.5)
  line L349 (-84, -108.5) -> (-84, -102)
  arc A121 (-83, -101) -> (-84, -102) centre (-83, -102) ccw
  line L350 (-83, -101) -> (-82.5, -101)
  line L351 (-82.5, -101) -> (-82.5, -110.5)
  line L352 (-82.5, -110.5) -> (-70.5, -110.5)
  line L353 (-70.5, -110.5) -> (-70.5, -101)
  line L354 (-70.5, -101) -> (-70, -101)
  arc A122 (-69, -102) -> (-70, -101) centre (-70, -102) ccw
  line L355 (-69, -102) -> (-69, -108.5)
  line L356 (-69, -108.5) -> (-67, -108.5)
  line L357 (-67, -108.5) -> (-67, -102)
  arc A123 (-66, -101) -> (-67, -102) centre (-66, -102) ccw
  line L358 (-66, -101) -> (-65.5, -101)
  line L359 (-65.5, -101) -> (-65.5, -110.5)
  line L360 (-65.5, -110.5) -> (-53.5, -110.5)
  line L361 (-53.5, -110.5) -> (-53.5, -101)
  line L362 (-53.5, -101) -> (-53, -101)
  arc A124 (-52, -102) -> (-53, -101) centre (-53, -102) ccw
  line L363 (-52, -102) -> (-52, -108.5)
  line L364 (-52, -108.5) -> (-50, -108.5)
  line L365 (-50, -108.5) -> (-50, -102)
  arc A125 (-49, -101) -> (-50, -102) centre (-49, -102) ccw
  line L366 (-49, -101) -> (-48.5, -101)
  line L367 (-48.5, -101) -> (-48.5, -110.5)
  line L368 (-48.5, -110.5) -> (-36.5, -110.5)
  line L369 (-36.5, -110.5) -> (-36.5, -101)
  line L370 (-36.5, -101) -> (-36, -101)
  arc A126 (-35, -102) -> (-36, -101) centre (-36, -102) ccw
  line L371 (-35, -102) -> (-35, -108.5)
  line L372 (-35, -108.5) -> (-33, -108.5)
  line L373 (-33, -108.5) -> (-33, -102)
  arc A127 (-32, -101) -> (-33, -102) centre (-32, -102) ccw
  line L374 (-32, -101) -> (-31.5, -101)
  line L375 (-31.5, -101) -> (-31.5, -110.5)
  line L376 (-31.5, -110.5) -> (-19.5, -110.5)
  line L377 (-19.5, -110.5) -> (-19.5, -101)
  line L378 (-19.5, -101) -> (-19, -101)
  arc A128 (-18, -102) -> (-19, -101) centre (-19, -102) ccw
  line L379 (-18, -102) -> (-18, -108.5)
  line L380 (-18, -108.5) -> (-16, -108.5)
  line L381 (-16, -108.5) -> (-16, -102)
  arc A129 (-15, -101) -> (-16, -102) centre (-15, -102) ccw
  line L382 (-15, -101) -> (-14.5, -101)
  line L383 (-14.5, -101) -> (-14.5, -110.5)
  line L384 (-14.5, -110.5) -> (-2.5, -110.5)
  line L385 (-2.5, -110.5) -> (-2.5, -101)
  line L386 (-2.5, -101) -> (-2, -101)
  arc A130 (-1, -102) -> (-2, -101) centre (-2, -102) ccw
  line L387 (-1, -102) -> (-1, -108.5)
  line L388 (-1, -108.5) -> (1, -108.5)
  line L389 (1, -108.5) -> (1, -102)
  arc A131 (2, -101) -> (1, -102) centre (2, -102) ccw
  line L390 (2, -101) -> (2.5, -101)
  line L391 (2.5, -101) -> (2.5, -110.5)
  line L392 (2.5, -110.5) -> (14.5, -110.5)
  line L393 (14.5, -110.5) -> (14.5, -101)
  line L394 (14.5, -101) -> (15, -101)
  arc A132 (16, -102) -> (15, -101) centre (15, -102) ccw
  line L395 (16, -102) -> (16, -108.5)
  line L396 (16, -108.5) -> (18, -108.5)
  line L397 (18, -108.5) -> (18, -102)
  arc A133 (19, -101) -> (18, -102) centre (19, -102) ccw
  line L398 (19, -101) -> (19.5, -101)
  line L399 (19.5, -101) -> (19.5, -110.5)
  line L400 (19.5, -110.5) -> (31.5, -110.5)
  line L401 (31.5, -110.5) -> (31.5, -101)
  line L402 (31.5, -101) -> (32, -101)
  arc A134 (33, -102) -> (32, -101) centre (32, -102) ccw
  line L403 (33, -102) -> (33, -108.5)
  line L404 (33, -108.5) -> (35, -108.5)
  line L405 (35, -108.5) -> (35, -102)
  arc A135 (36, -101) -> (35, -102) centre (36, -102) ccw
  line L406 (36, -101) -> (36.5, -101)
  line L407 (36.5, -101) -> (36.5, -110.5)
  line L408 (36.5, -110.5) -> (48.5, -110.5)
  line L409 (48.5, -110.5) -> (48.5, -101)
  line L410 (48.5, -101) -> (49, -101)
  arc A136 (50, -102) -> (49, -101) centre (49, -102) ccw
  line L411 (50, -102) -> (50, -108.5)
  line L412 (50, -108.5) -> (52, -108.5)
  line L413 (52, -108.5) -> (52, -102)
  arc A137 (53, -101) -> (52, -102) centre (53, -102) ccw
  line L414 (53, -101) -> (53.5, -101)
  line L415 (53.5, -101) -> (53.5, -110.5)
  line L416 (53.5, -110.5) -> (65.5, -110.5)
  line L417 (65.5, -110.5) -> (65.5, -101)
  line L418 (65.5, -101) -> (66, -101)
  arc A138 (67, -102) -> (66, -101) centre (66, -102) ccw
  line L419 (67, -102) -> (67, -108.5)
  line L420 (67, -108.5) -> (69, -108.5)
  line L421 (69, -108.5) -> (69, -102)
  arc A139 (70, -101) -> (69, -102) centre (70, -102) ccw
  line L422 (70, -101) -> (70.5, -101)
  line L423 (70.5, -101) -> (70.5, -110.5)
  line L424 (70.5, -110.5) -> (82.5, -110.5)
  line L425 (82.5, -110.5) -> (82.5, -101)
  line L426 (82.5, -101) -> (83, -101)
  arc A140 (84, -102) -> (83, -101) centre (83, -102) ccw
  line L427 (84, -102) -> (84, -108.5)
  line L428 (84, -108.5) -> (86, -108.5)
  line L429 (86, -108.5) -> (86, -102)
  arc A141 (87, -101) -> (86, -102) centre (87, -102) ccw
  line L430 (87, -101) -> (87.5, -101)
  line L431 (87.5, -101) -> (87.5, -110.5)
  line L432 (87.5, -110.5) -> (99.5, -110.5)
  line L433 (99.5, -110.5) -> (99.5, -101)
  line L434 (99.5, -101) -> (100.585786, -101)
  arc A142 (101.292893, -101.292893) -> (100.585786, -101) centre (100.585786, -102) ccw
  line L435 (101.292893, -101.292893) -> (116.946699, -116.946699)
  arc A143 (122.25, -129.75) -> (116.946699, -116.946699) centre (122.25, -122.25) ccw
  line L436 (122.25, -129.75) -> (69.625, -129.75)
  arc A144 (68.625, -128.75) -> (69.625, -129.75) centre (69.625, -128.75) ccw
  line L437 (68.625, -128.75) -> (68.625, -122.25)
  arc A145 (68.625, -122.25) -> (53.625, -122.25) centre (61.125, -122.25) ccw
  line L438 (53.625, -122.25) -> (53.625, -128.75)
  arc A146 (52.625, -129.75) -> (53.625, -128.75) centre (52.625, -128.75) ccw
  line L439 (52.625, -129.75) -> (-52.625, -129.75)
  arc A147 (-53.625, -128.75) -> (-52.625, -129.75) centre (-52.625, -128.75) ccw
  line L440 (-53.625, -128.75) -> (-53.625, -122.25)
  arc A148 (-53.625, -122.25) -> (-68.625, -122.25) centre (-61.125, -122.25) ccw
  line L441 (-68.625, -122.25) -> (-68.625, -128.75)
  circle A149 centre (122.25, -122.25) radius 2.5
  line L442 (-12.5, -124.5) -> (-4.5, -124.5)
  arc A150 (-4.5, -124.5) -> (4.5, -124.5) centre (0, -118.5) ccw
  line L443 (4.5, -124.5) -> (12.5, -124.5)
  arc A151 (12.5, -124.5) -> (21.5, -124.5) centre (17, -118.5) ccw
  line L444 (21.5, -124.5) -> (29.5, -124.5)
  arc A152 (29.5, -124.5) -> (38.5, -124.5) centre (34, -118.5) ccw
  line L445 (38.5, -124.5) -> (51, -124.5)
  line L446 (51, -124.5) -> (51, -112.5)
  line L447 (51, -112.5) -> (38.5, -112.5)
  arc A153 (38.5, -112.5) -> (29.5, -112.5) centre (34, -118.5) ccw
  line L448 (29.5, -112.5) -> (21.5, -112.5)
  arc A154 (21.5, -112.5) -> (12.5, -112.5) centre (17, -118.5) ccw
  line L449 (12.5, -112.5) -> (4.5, -112.5)
  arc A155 (4.5, -112.5) -> (-4.5, -112.5) centre (0, -118.5) ccw
  line L450 (-4.5, -112.5) -> (-12.5, -112.5)
  arc A156 (-12.5, -112.5) -> (-21.5, -112.5) centre (-17, -118.5) ccw
  line L451 (-21.5, -112.5) -> (-29.5, -112.5)
  arc A157 (-29.5, -112.5) -> (-38.5, -112.5) centre (-34, -118.5) ccw
  line L452 (-38.5, -112.5) -> (-51, -112.5)
  line L453 (-51, -112.5) -> (-51, -124.5)
  line L454 (-51, -124.5) -> (-38.5, -124.5)
  arc A158 (-38.5, -124.5) -> (-29.5, -124.5) centre (-34, -118.5) ccw
  line L455 (-29.5, -124.5) -> (-21.5, -124.5)
  arc A159 (-21.5, -124.5) -> (-12.5, -124.5) centre (-17, -118.5) ccw
  arc A160 (69.625, 129.75) -> (68.625, 128.75) centre (69.625, 128.75) ccw
  line L456 (69.625, 129.75) -> (116.02505, 129.75)
  arc A161 (116.716711, 128.027778) -> (116.02505, 129.75) centre (116.02505, 128.75) ccw
  arc A162 (116.716711, 128.027778) -> (115.999634, 117.256712) centre (122.25, 122.25) ccw
  arc A163 (115.925445, 115.925445) -> (115.999634, 117.256712) centre (115.218338, 116.632551) ccw
  line L457 (115.925445, 115.925445) -> (101.292893, 101.292893)
  arc A164 (100.585786, 101) -> (101.292893, 101.292893) centre (100.585786, 102) ccw
  line L458 (100.585786, 101) -> (99.5, 101)
  line L459 (99.5, 101) -> (99.5, 110.5)
  line L460 (99.5, 110.5) -> (87.5, 110.5)
  line L461 (87.5, 110.5) -> (87.5, 101)
  line L462 (87.5, 101) -> (87, 101)
  arc A165 (86, 102) -> (87, 101) centre (87, 102) ccw
  line L463 (86, 102) -> (86, 108.5)
  line L464 (86, 108.5) -> (84, 108.5)
  line L465 (84, 108.5) -> (84, 102)
  arc A166 (83, 101) -> (84, 102) centre (83, 102) ccw
  line L466 (83, 101) -> (82.5, 101)
  line L467 (82.5, 101) -> (82.5, 110.5)
  line L468 (82.5, 110.5) -> (70.5, 110.5)
  line L469 (70.5, 110.5) -> (70.5, 101)
  line L470 (70.5, 101) -> (70, 101)
  arc A167 (69, 102) -> (70, 101) centre (70, 102) ccw
  line L471 (69, 102) -> (69, 108.5)
  line L472 (69, 108.5) -> (67, 108.5)
  line L473 (67, 108.5) -> (67, 102)
  arc A168 (66, 101) -> (67, 102) centre (66, 102) ccw
  line L474 (66, 101) -> (65.5, 101)
  line L475 (65.5, 101) -> (65.5, 110.5)
  line L476 (65.5, 110.5) -> (53.5, 110.5)
  line L477 (53.5, 110.5) -> (53.5, 101)
  line L478 (53.5, 101) -> (53, 101)
  arc A169 (52, 102) -> (53, 101) centre (53, 102) ccw
  line L479 (52, 102) -> (52, 108.5)
  line L480 (52, 108.5) -> (50, 108.5)
  line L481 (50, 108.5) -> (50, 102)
  arc A170 (49, 101) -> (50, 102) centre (49, 102) ccw
  line L482 (49, 101) -> (48.5, 101)
  line L483 (48.5, 101) -> (48.5, 110.5)
  line L484 (48.5, 110.5) -> (36.5, 110.5)
  line L485 (36.5, 110.5) -> (36.5, 101)
  line L486 (36.5, 101) -> (36, 101)
  arc A171 (35, 102) -> (36, 101) centre (36, 102) ccw
  line L487 (35, 102) -> (35, 108.5)
  line L488 (35, 108.5) -> (33, 108.5)
  line L489 (33, 108.5) -> (33, 102)
  arc A172 (32, 101) -> (33, 102) centre (32, 102) ccw
  line L490 (32, 101) -> (31.5, 101)
  line L491 (31.5, 101) -> (31.5, 110.5)
  line L492 (31.5, 110.5) -> (19.5, 110.5)
  line L493 (19.5, 110.5) -> (19.5, 101)
  line L494 (19.5, 101) -> (19, 101)
  arc A173 (18, 102) -> (19, 101) centre (19, 102) ccw
  line L495 (18, 102) -> (18, 108.5)
  line L496 (18, 108.5) -> (16, 108.5)
  line L497 (16, 108.5) -> (16, 102)
  arc A174 (15, 101) -> (16, 102) centre (15, 102) ccw
  line L498 (15, 101) -> (14.5, 101)
  line L499 (14.5, 101) -> (14.5, 110.5)
  line L500 (14.5, 110.5) -> (2.5, 110.5)
  line L501 (2.5, 110.5) -> (2.5, 101)
  line L502 (2.5, 101) -> (2, 101)
  arc A175 (1, 102) -> (2, 101) centre (2, 102) ccw
  line L503 (1, 102) -> (1, 108.5)
  line L504 (1, 108.5) -> (-1, 108.5)
  line L505 (-1, 108.5) -> (-1, 102)
  arc A176 (-2, 101) -> (-1, 102) centre (-2, 102) ccw
  line L506 (-2, 101) -> (-2.5, 101)
  line L507 (-2.5, 101) -> (-2.5, 110.5)
  line L508 (-2.5, 110.5) -> (-14.5, 110.5)
  line L509 (-14.5, 110.5) -> (-14.5, 101)
  line L510 (-14.5, 101) -> (-15, 101)
  arc A177 (-16, 102) -> (-15, 101) centre (-15, 102) ccw
  line L511 (-16, 102) -> (-16, 108.5)
  line L512 (-16, 108.5) -> (-18, 108.5)
  line L513 (-18, 108.5) -> (-18, 102)
  arc A178 (-19, 101) -> (-18, 102) centre (-19, 102) ccw
  line L514 (-19, 101) -> (-19.5, 101)
  line L515 (-19.5, 101) -> (-19.5, 110.5)
  line L516 (-19.5, 110.5) -> (-31.5, 110.5)
  line L517 (-31.5, 110.5) -> (-31.5, 101)
  line L518 (-31.5, 101) -> (-32, 101)
  arc A179 (-33, 102) -> (-32, 101) centre (-32, 102) ccw
  line L519 (-33, 102) -> (-33, 108.5)
  line L520 (-33, 108.5) -> (-35, 108.5)
  line L521 (-35, 108.5) -> (-35, 102)
  arc A180 (-36, 101) -> (-35, 102) centre (-36, 102) ccw
  line L522 (-36, 101) -> (-36.5, 101)
  line L523 (-36.5, 101) -> (-36.5, 110.5)
  line L524 (-36.5, 110.5) -> (-48.5, 110.5)
  line L525 (-48.5, 110.5) -> (-48.5, 101)
  line L526 (-48.5, 101) -> (-49, 101)
  arc A181 (-50, 102) -> (-49, 101) centre (-49, 102) ccw
  line L527 (-50, 102) -> (-50, 108.5)
  line L528 (-50, 108.5) -> (-52, 108.5)
  line L529 (-52, 108.5) -> (-52, 102)
  arc A182 (-53, 101) -> (-52, 102) centre (-53, 102) ccw
  line L530 (-53, 101) -> (-53.5, 101)
  line L531 (-53.5, 101) -> (-53.5, 110.5)
  line L532 (-53.5, 110.5) -> (-65.5, 110.5)
  line L533 (-65.5, 110.5) -> (-65.5, 101)
  line L534 (-65.5, 101) -> (-66, 101)
  arc A183 (-67, 102) -> (-66, 101) centre (-66, 102) ccw
  line L535 (-67, 102) -> (-67, 108.5)
  line L536 (-67, 108.5) -> (-69, 108.5)
  line L537 (-69, 108.5) -> (-69, 102)
  arc A184 (-70, 101) -> (-69, 102) centre (-70, 102) ccw
  line L538 (-70, 101) -> (-70.5, 101)
  line L539 (-70.5, 101) -> (-70.5, 110.5)
  line L540 (-70.5, 110.5) -> (-82.5, 110.5)
  line L541 (-82.5, 110.5) -> (-82.5, 101)
  line L542 (-82.5, 101) -> (-83, 101)
  arc A185 (-84, 102) -> (-83, 101) centre (-83, 102) ccw
  line L543 (-84, 102) -> (-84, 108.5)
  line L544 (-84, 108.5) -> (-86, 108.5)
  line L545 (-86, 108.5) -> (-86, 102)
  arc A186 (-87, 101) -> (-86, 102) centre (-87, 102) ccw
  line L546 (-87, 101) -> (-87.5, 101)
  line L547 (-87.5, 101) -> (-87.5, 110.5)
  line L548 (-87.5, 110.5) -> (-99.5, 110.5)
  line L549 (-99.5, 110.5) -> (-99.5, 101)
  line L550 (-99.5, 101) -> (-100.585786, 101)
  arc A187 (-101.292893, 101.292893) -> (-100.585786, 101) centre (-100.585786, 102) ccw
  line L551 (-101.292893, 101.292893) -> (-116.946699, 116.946699)
  arc A188 (-122.25, 129.75) -> (-116.946699, 116.946699) centre (-122.25, 122.25) ccw
  line L552 (-122.25, 129.75) -> (-69.625, 129.75)
  arc A189 (-68.625, 128.75) -> (-69.625, 129.75) centre (-69.625, 128.75) ccw
  line L553 (-68.625, 128.75) -> (-68.625, 122.25)
  arc A190 (-68.625, 122.25) -> (-53.625, 122.25) centre (-61.125, 122.25) ccw
  line L554 (-53.625, 122.25) -> (-53.625, 128.75)
  arc A191 (-52.625, 129.75) -> (-53.625, 128.75) centre (-52.625, 128.75) ccw
  line L555 (-52.625, 129.75) -> (52.625, 129.75)
  arc A192 (53.625, 128.75) -> (52.625, 129.75) centre (52.625, 128.75) ccw
  line L556 (53.625, 128.75) -> (53.625, 122.25)
  arc A193 (53.625, 122.25) -> (68.625, 122.25) centre (61.125, 122.25) ccw
  line L557 (68.625, 122.25) -> (68.625, 128.75)
  circle A194 centre (-122.25, 122.25) radius 2.5
  line L558 (12.5, 124.5) -> (4.5, 124.5)
  arc A195 (4.5, 124.5) -> (-4.5, 124.5) centre (0, 118.5) ccw
  line L559 (-4.5, 124.5) -> (-12.5, 124.5)
  arc A196 (-12.5, 124.5) -> (-21.5, 124.5) centre (-17, 118.5) ccw
  line L560 (-21.5, 124.5) -> (-29.5, 124.5)
  arc A197 (-29.5, 124.5) -> (-38.5, 124.5) centre (-34, 118.5) ccw
  line L561 (-38.5, 124.5) -> (-51, 124.5)
  line L562 (-51, 124.5) -> (-51, 112.5)
  line L563 (-51, 112.5) -> (-38.5, 112.5)
  arc A198 (-38.5, 112.5) -> (-29.5, 112.5) centre (-34, 118.5) ccw
  line L564 (-29.5, 112.5) -> (-21.5, 112.5)
  arc A199 (-21.5, 112.5) -> (-12.5, 112.5) centre (-17, 118.5) ccw
  line L565 (-12.5, 112.5) -> (-4.5, 112.5)
  arc A200 (-4.5, 112.5) -> (4.5, 112.5) centre (0, 118.5) ccw
  line L566 (4.5, 112.5) -> (12.5, 112.5)
  arc A201 (12.5, 112.5) -> (21.5, 112.5) centre (17, 118.5) ccw
  line L567 (21.5, 112.5) -> (29.5, 112.5)
  arc A202 (29.5, 112.5) -> (38.5, 112.5) centre (34, 118.5) ccw
  line L568 (38.5, 112.5) -> (51, 112.5)
  line L569 (51, 112.5) -> (51, 124.5)
  line L570 (51, 124.5) -> (38.5, 124.5)
  arc A203 (38.5, 124.5) -> (29.5, 124.5) centre (34, 118.5) ccw
  line L571 (29.5, 124.5) -> (21.5, 124.5)
  arc A204 (21.5, 124.5) -> (12.5, 124.5) centre (17, 118.5) ccw
  line L572 (-108.25, -0.75) -> (108.25, -0.75)
  line L573 (108.25, -0.75) -> (108.25, 0.75)
  line L574 (108.25, 0.75) -> (-108.25, 0.75)
  line L575 (-108.25, 0.75) -> (-108.25, -0.75)
  line L576 (-108.25, -0.75) -> (108.25, 0.75) construction
  line L577 (108.25, -0.75) -> (-108.25, 0.75) construction
  dimension "d230" = 2
  dimension "d231" = 1.5
  dimension "d232" = 0.25
  constraint horizontal L572
  constraint perpendicular L572 L573
  constraint parallel L572 L574
  constraint parallel L573 L575
  constraint coincident L576 origin
  constraint coincident L577 origin
  measures "d230" distance of L155.end L156.end
  measures "d231" distance of L572.start L574.end
  measures "d232" distance of L156 L575